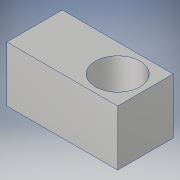
# Autodesk Inventor part: sheild stop
Saved by Autodesk Inventor 2018 (Build 220112000, 112)
## iProperties
Created: 2018-10-14
Part Number: sheild stop
Material: Aluminum 6061
Document SubType Name: Modeling
Designer: freyja
Mass: 1.38266 g
Surface Area: 4.03225 cm^2
Volume: 0.512096 cm^3
Density: 2.7 g/cm^3
Appearance: Aluminum - Flat
Author: freyja
Autodesk Inventor part; units mm, degrees
note: some values were not read from the file. Chosen so that the rebuilt part matches the saved one: direction of "Hole1".
ref_plane "YZ Plane" through (0, 0, 0) normal (1, 0, 0) x (0, 1, 0)
ref_plane "XZ Plane" through (0, 0, 0) normal (0, 1, 0) x (-1, 0, 0)
ref_plane "XY Plane" through (0, 0, 0) normal (0, 0, 1) x (1, 0, 0)
sketch "Sketch1" plane through (0, 0, 0) normal (0, 1, 0) x (-1, 0, 0)
  line L0 (-6.35, -3.175) -> (6.35, -3.175)
  line L1 (6.35, -3.175) -> (6.35, 3.175)
  line L2 (6.35, 3.175) -> (-6.35, 3.175)
  line L3 (-6.35, 3.175) -> (-6.35, -3.175)
  line L4 (-6.35, -3.175) -> (6.35, 3.175) construction
  line L5 (6.35, -3.175) -> (-6.35, 3.175) construction
  point P0 (0, 0)
  dimension "d0" = 12.7
  dimension "d1" = 6.35
  constraints: 12 end point, 2 midpoint, 2 parallel, 1 horizontal, 1 perpendicular
  measures "d0" distance of L2.end L1.end
  measures "d1" distance of L1.end L0.end
extrude "Extrusion1" add sketch "Sketch1" along normal blind 6.35
sketch "Sketch2" plane through (0, 6.35, 0) normal (0, 1, 0) x (1, 0, 0)
  line L0 (0, 0) -> (3.175, 0)
  dimension "d4" = 3.175
  constraints: 2 end point, 1 horizontal
  measures "d4" distance of L0.start L0.end
hole "Hole1" at (3.175, 6.35, 0) direction (0, -1, 0) diameter 5.1054 end up to surface clearance for "Flat Head Machine Screw (82)" size "#10" standard "Ansi Unified Screw Threads"
body "Solid1"
